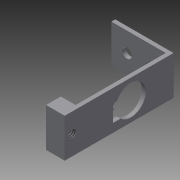
# Autodesk Inventor part: 000208
Saved by Autodesk Inventor 2015 (Build 190159000, 159)
## iProperties
Created: 2015-05-29
Part Number: 000208
Material: Generic
Document SubType Name: Modeling
Designer: Wesley
Density: 1 g/cm^3
Appearance: Default
Author: Wesley
Autodesk Inventor part; units mm, degrees
ref_plane "YZ Plane" through (0, 0, 0) normal (1, 0, 0) x (0, 1, 0)
ref_plane "XZ Plane" through (0, 0, 0) normal (0, 1, 0) x (-1, 0, 0)
ref_plane "XY Plane" through (0, 0, 0) normal (0, 0, 1) x (1, 0, 0)
sketch "Sketch1" plane through (0, 0, 0) normal (0, 0, 1) x (1, 0, 0)
  line L0 (0, 0) -> (19.05, 0)
  line L1 (19.05, 0) -> (19.05, 12.7)
  line L2 (19.05, 12.7) -> (0, 12.7)
  line L3 (0, 12.7) -> (0, 0)
  circle A0 centre (5.08, 6.35) radius 1.5875
  circle A1 centre (12.7, 6.35) radius 1.5875
  dimension "d0" = 12.7
  dimension "d1" = 19.05
  dimension "d2" = 3.175
  dimension "d3" = 3.175
  dimension "d4" = 6.35
  dimension "d5" = 5.08
  dimension "d6" = 7.62
  constraints: 8 end point, 2 centre point, 2 parallel, 1 horizontal, 1 horizontal alignment, 1 perpendicular
  measures "d0" distance of L2.end L0.start
  measures "d1" distance of L0.start L0.end
  measures "d2" diameter of A0
  measures "d3" diameter of A1
  measures "d4" distance from line of L0 A0.centre
  measures "d5" distance from line of L3 A0.centre
  measures "d6" distance of A0.centre A1.centre
extrude "Extrusion1" add sketch "Sketch1" along normal blind 1.27
sketch "Sketch2" plane through (0, 0, 1.27) normal (0, 0, 1) x (1, 0, 0)
  line L0 (19.05, 12.7) -> (0, 12.7) projected
  line L1 (19.05, 0) -> (17.78, 0)
  line L2 (17.78, 0) -> (17.78, 12.7)
  line L3 (17.78, 12.7) -> (19.05, 12.7)
  line L4 (19.05, 12.7) -> (19.05, 0)
  point P0 (0, 0)
  dimension "d9" = 1.27
  constraints: 8 end point, 2 parallel, 1 horizontal, 1 perpendicular, 1 point on line
  measures "d9" distance of L2.end L3.end
extrude "Extrusion2" add sketch "Sketch2" along normal blind 34.29
sketch "Sketch3" plane through (17.78, 0, 1.27) normal (-1, 0, 0) x (0, 0, 1)
  line L0 (0, 12.7) -> (0, 0) projected
  line L1 (0, 12.7) -> (34.29, 12.7) projected
  arc A0 (17.2142, 8.2614) -> (16.0744, 2.794) centre (12.7, 6.35) ccw
  line L2 (17.6022, 6.35) -> (18.5128, 6.35)
  line L3 (18.5128, 6.35) -> (18.5128, 2.794)
  line L4 (18.5128, 2.794) -> (16.0744, 2.794)
  line L5 (16.0744, 2.794) -> (16.0744, 6.35)
  arc A1 (17.8973, 6.35) -> (17.2142, 8.2614) centre (17.5113, 7.2898) ccw
  point P0 (-1.27, 0)
  point P1 (17.2936, 6.35)
  dimension "d21" = 9.8044
  dimension "d22" = 12.7
  dimension "d23" = 6.35
  dimension "d24" = 3.556
  dimension "d25" = 2.4384
  dimension "d26" = 2.032
  dimension "d27" = 0.9398
  dimension "d28" = 3.556
  constraints: 8 end point, 5 point on circle, 2 centre point, 2 parallel, 2 point on line, 1 horizontal, 1 horizontal alignment, 1 perpendicular
  measures "d21" diameter of A0
  measures "d22" distance from line of A0.centre L0
  measures "d23" distance from line of L1 A0.centre
  measures "d24" distance of L4.end L5.end
  measures "d25" distance of L3.end L4.end
  measures "d26" diameter of A1
  measures "d27" distance from line of A1.centre L2
  measures "d28" distance of L2.end L3.end
extrude "Extrusion3" cut sketch "Sketch3" against normal blind 25.4
sketch "Sketch4" plane through (17.78, 0, 1.27) normal (-1, 0, 0) x (0, 0, 1)
  line L0 (34.29, 12.7) -> (29.464, 12.7)
  line L1 (29.464, 12.7) -> (29.464, 0)
  line L2 (29.464, 0) -> (34.29, 0)
  line L3 (34.29, 0) -> (34.29, 12.7)
  arc A0 (17.2142, 8.2614) -> (16.0744, 2.794) centre (12.7, 6.35) ccw projected
  line L4 (0, 0) -> (34.29, 0) projected
  point P0 (-1.27, 0)
  point P1 (31.877, 0)
  dimension "d29" = 16.764
  constraints: 8 end point, 2 parallel, 1 horizontal, 1 midpoint, 1 perpendicular, 1 point on line
  measures "d29" distance from line of L1 A0.centre
extrude "Extrusion4" add sketch "Sketch4" along normal blind 4.826
sketch "Sketch5" plane through (12.954, 0, 1.27) normal (-1, 0, 0) x (0, 0, 1)
  line L0 (34.29, 12.7) -> (29.464, 12.7) projected
  line L1 (29.464, 12.7) -> (29.464, 0) projected
  line L2 (29.464, 0) -> (34.29, 0) projected
  line L3 (34.29, 0) -> (34.29, 12.7) projected
  point P0 (-1.27, 0)
  point P1 (31.8008, 6.35)
  dimension "d33" = 4.826
  dimension "d35" = 12.7
  dimension "d38" = 6.35
  dimension "d46" = 2.3368
  measures "d33" distance of L0.start L0.end
  measures "d35" distance of L2.end L0.start
  measures "d38" distance from line of L2 point (31.801, 6.35)
  measures "d46" distance from line of L1 point (31.801, 6.35)
hole "Hole1" at (12.954, 6.35, 33.0708) direction (1, 0, 0) diameter 2.4892 end through all
body "Solid1"
